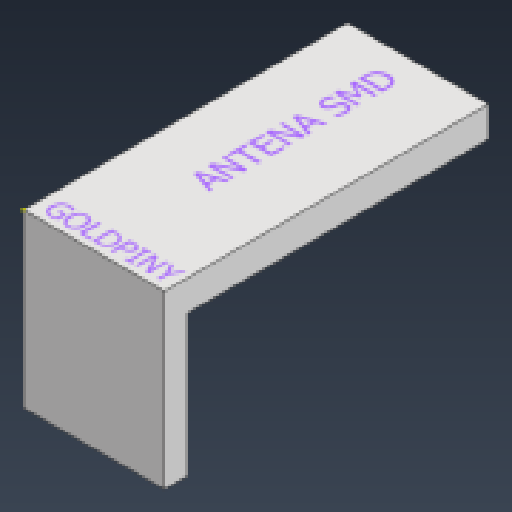
# Autodesk Inventor part: controller_reveiver
Saved by Autodesk Inventor 2023 (Build 270158000, 158)
## iProperties
Created: 2025-12-27
Part Number: controller_reveiver
Material: Generic
Document SubType Name: Modeling
Designer: szymo
Density: 1 g/cm^3
Appearance: Default
Author: szymo
Autodesk Inventor part; units mm, degrees
ref_plane "YZ Plane" through (0, 0, 0) normal (1, 0, 0) x (0, 1, 0)
ref_plane "XZ Plane" through (0, 0, 0) normal (0, 1, 0) x (-1, 0, 0)
ref_plane "XY Plane" through (0, 0, 0) normal (0, 0, 1) x (1, 0, 0)
sketch "Sketch1" plane through (0, 0, 0) normal (0, 1, 0) x (-1, 0, 0)
  line L0 (0, 0) -> (-18.5, 0)
  line L1 (-18.5, 0) -> (-18.5, -42.5)
  line L2 (-18.5, -42.5) -> (0, -42.5)
  line L3 (0, -42.5) -> (0, 0)
  dimension "d0" = 18.5
  dimension "d1" = 42.5
  constraints: 8 end point, 2 parallel, 1 horizontal, 1 perpendicular
  measures "d0" distance of L2.end L1.end
  measures "d1" distance of L1.end L0.end
extrude "Extrusion1" add sketch "Sketch1" along normal blind 4
sketch "Sketch2" plane through (0, 0, 0) normal (0, -1, 0) x (1, 0, 0)
  line L0 (0, -42.5) -> (0, 0) projected
  line L1 (18.5, 0) -> (18.5, -42.5) projected
  line L2 (0, 0) -> (18.5, 0)
  line L3 (18.5, 0) -> (18.5, -3)
  line L4 (18.5, -3) -> (0, -3)
  line L5 (0, -3) -> (0, 0)
  dimension "d4" = 3
  constraints: 8 end point, 2 parallel, 1 horizontal, 1 perpendicular, 1 point on line
  measures "d4" distance of L2.end L3.end
extrude "Extrusion2" add sketch "Sketch2" along normal blind 18.5
sketch "Sketch3" plane through (0, 4, 0) normal (0, 1, 0) x (1, 0, 0)
  line L0 (1.2509, 3.5794) -> (17.7774, 3.5794) construction
  line L1 (17.7774, 3.5794) -> (17.7774, 0.9324) construction
  line L2 (17.7774, 0.9324) -> (1.2509, 0.9324) construction
  line L3 (1.2509, 0.9324) -> (1.2509, 3.5794) construction
  line L4 (7.0482, 14.2862) -> (7.0482, 39.4285) construction
  line L5 (7.0482, 39.4285) -> (10.2049, 39.4285) construction
  line L6 (10.2049, 39.4285) -> (10.2049, 14.2862) construction
  line L7 (10.2049, 14.2862) -> (7.0482, 14.2862) construction
  point P0 (0, 0)
  dimension "d2" = 4
  dimension "d3" = 0
  constraints: 4 other
body "Solid1"
